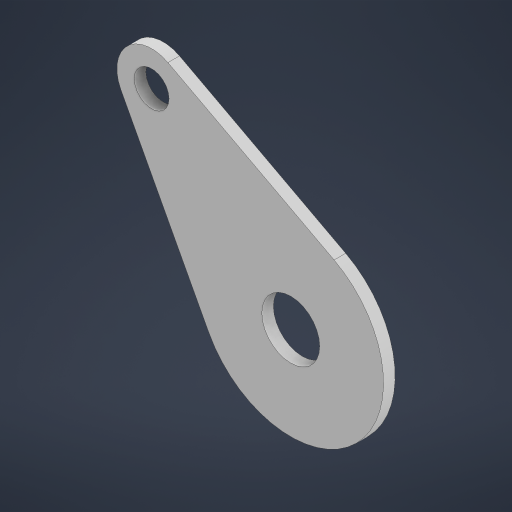
# Autodesk Inventor part: pto
Saved by Autodesk Inventor 2024 (Build 280153000, 153)
## iProperties
Created: 2023-11-19
Part Number: pto
Material: Generic
Document SubType Name: Modeling
Designer: macbook
Density: 1 g/cm^3
Appearance: Default
Author: macbook
Autodesk Inventor part; units mm, degrees
ref_plane "YZ Plane" through (0, 0, 0) normal (1, 0, 0) x (0, 1, 0)
ref_plane "XZ Plane" through (0, 0, 0) normal (0, 1, 0) x (-1, 0, 0)
ref_plane "XY Plane" through (0, 0, 0) normal (0, 0, 1) x (1, 0, 0)
sketch "Sketch1" plane through (0, 0, 0) normal (0, 0, 1) x (1, 0, 0)
  line L0 (0, 0) -> (0, -19.05) construction
  line L1 (0, -19.05) -> (19.05, -19.05) construction
  circle A0 centre (0, 0) radius 2.3813
  circle A1 centre (19.05, -19.05) radius 3.9687
  circle A2 centre (0, 0) radius 4.7625
  circle A3 centre (19.05, -19.05) radius 12.7
  line L2 (0, 0) -> (19.05, -19.05) construction
  line L3 (-4.3763, -1.912) -> (11.0982, -31.1817)
  line L4 (1.2997, 4.7) -> (30.5694, -10.7745)
  point P0 (7.7583, -1.6771)
  point P1 (-4.2103, -2.2259)
  point P2 (7.8225, -24.9858)
  point P3 (24.9858, -7.8225)
  point P4 (2.2259, 4.2103)
  dimension "d0" = 19.05
  dimension "d1" = 19.05
  dimension "d2" = 4.7625
  dimension "d3" = 7.9375
  dimension "d4" = 9.525
  dimension "d5" = 25.4
  constraints: 10 end point, 4 centre point, 4 coincident, 4 tangent, 1 horizontal, 1 vertical
  measures "d0" distance of L0.start L0.end
  measures "d1" distance of L0.end L1.end
  measures "d2" diameter of A0
  measures "d3" diameter of A1
  measures "d4" diameter of A2
  measures "d5" diameter of A3
extrude "Extrusion1" add sketch "Sketch1" along normal blind 1.5875
body "Solid1"
